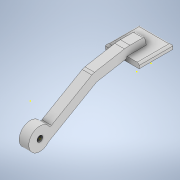
# Autodesk Inventor part: moving gripper
Saved by Autodesk Inventor 2021 (Build 250183000, 183)
## iProperties
Created: 2021-01-30
Part Number: moving gripper
Material: Generic
Document SubType Name: Modeling
Designer: josep
Density: 1 g/cm^3
Appearance: Default
Author: josep
Autodesk Inventor part; units mm, degrees
ref_plane "YZ Plane" through (0, 0, 0) normal (1, 0, 0) x (0, 1, 0)
ref_plane "XZ Plane" through (0, 0, 0) normal (0, 1, 0) x (-1, 0, 0)
ref_plane "XY Plane" through (0, 0, 0) normal (0, 0, 1) x (1, 0, 0)
sketch "Sketch1" plane through (0, 0, 0) normal (1, 0, 0) x (0, 1, 0)
  circle A0 centre (0, 0) radius 11.5
  line L0 (0, -11.5) -> (51.956, -11.5) construction
  line L1 (17.8954, -32.4957) -> (5.0882, -10.3131)
  line L2 (9.2351, -37.4957) -> (-7.2673, -8.9127)
  line L3 (9.2351, -37.4957) -> (21.6479, -58.9952)
  line L4 (30.3081, -53.9952) -> (17.8954, -32.4957)
  line L5 (21.6479, -58.9952) -> (28.9335, -100.3138)
  line L6 (21.6479, -58.9952) -> (73.6039, -58.9952) construction
  line L7 (30.6699, -110.1619) -> (40.4125, -107.9075)
  line L8 (40.4125, -107.9075) -> (31.3905, -56.7409)
  line L9 (40.4125, -107.9075) -> (92.3685, -107.9075) construction
  arc A1 (31.3905, -56.7409) -> (30.3081, -53.9952) centre (21.6479, -58.9952) ccw
  line L10 (28.9335, -110.4681) -> (30.6699, -110.1619)
  line L11 (28.9335, -100.3138) -> (28.9335, -110.4681)
  dimension "d0" = 23
  dimension "d4" = 10
  dimension "d7" = 10
  dimension "d9" = 100
  constraints: 24 end point, 5 point on circle, 3 horizontal, 2 centre point, 2 point on line, 1 coincident, 1 equal length, 1 parallel, 1 vertical
  measures "d0" diameter of A0
  measures "d4" distance of L1.start L2.start
  measures "d7" distance of L7.start L7.end
  measures "d9" angle of L9 L8
extrude "Extrusion1" add sketch "Sketch1" along normal blind 10
sketch "Sketch2" plane through (0, 28.9335, -110.4681) normal (0, -1, 0) x (1, 0, 0)
  line L0 (10, 51.4729) -> (10, 10.1543) projected
  line L1 (10, 10.1543) -> (10, 0) projected
  line L2 (10, 10.1543) -> (10, 0)
  line L3 (0, 0) -> (10, 0) projected
  line L4 (10, 0) -> (0, 0)
  line L5 (0, 10.1543) -> (10, 10.1543) projected
  line L6 (0, 0) -> (0, 10.1543)
  line L7 (0, 10.1543) -> (10, 10.1543)
  point P0 (0, 110.4681)
  constraints: 8 end point, 3 collinear, 1 perpendicular
extrude "Extrusion2" add sketch "Sketch2" along normal blind 5
sketch "Sketch3" plane through (10, 28.9335, -110.4681) normal (0, 0, -1) x (-1, 0, 0)
  point P0 (10, -28.9335)
sketch "Sketch4" plane through (10, 28.9335, -110.4681) normal (0, 0, -1) x (-1, 0, 0)
  line L0 (0, 0) -> (0, 1.7365) projected
  line L1 (10, 0) -> (10, 1.7365) projected
  line L2 (0, 0) -> (10, 0)
  line L3 (10, 0) -> (10, -5)
  line L4 (10, -5) -> (0, -5)
  line L5 (0, -5) -> (0, 0)
  point P0 (10, -28.9335)
  constraints: 8 end point, 3 perpendicular, 1 horizontal
extrude "Extrusion3" add sketch "Sketch4" along normal blind 15
sketch "Sketch5" plane through (10, 28.9335, -125.4681) normal (0, 0, -1) x (-1, 0, 0)
  point P0 (10, -28.9335)
sketch "Sketch6" plane through (10, 28.9335, -125.4681) normal (0, 0, -1) x (-1, 0, 0)
  line L0 (10, 0) -> (0, 0) projected
  line L1 (0, 0) -> (10, 0)
  line L2 (10, -5) -> (10, 0) projected
  line L3 (10, 0) -> (10, -5)
  line L4 (0, -5) -> (10, -5) projected
  line L5 (10, -5) -> (0, -5)
  line L6 (0, 0) -> (0, -5) projected
  line L7 (0, -5) -> (0, 0)
  point P0 (10, -28.9335)
  constraints: 8 end point, 2 collinear, 1 horizontal, 1 perpendicular
extrude "Extrusion4" add sketch "Sketch6" against normal blind 35
sketch "Sketch7" plane through (10, 0, 0) normal (1, 0, 0) x (0, 0, -1)
  point P0 (0, 0)
sketch "Sketch8" plane through (10, 0, 0) normal (1, 0, 0) x (0, 0, -1)
  line L0 (125.4681, 28.9335) -> (125.4681, 23.9335) projected
  line L1 (125.4681, 28.9335) -> (125.4681, 23.9335)
  line L2 (90.4681, 23.9335) -> (90.4681, 27.1974) projected
  line L3 (125.4681, 23.9335) -> (90.4681, 23.9335)
  line L4 (90.4681, 23.9335) -> (90.4681, 28.9335)
  line L5 (110.4681, 28.9335) -> (125.4681, 28.9335) projected
  line L6 (90.4681, 28.9335) -> (125.4681, 28.9335)
  point P0 (0, 0)
  constraints: 8 end point, 2 perpendicular, 1 collinear, 1 vertical
extrude "Extrusion5" add sketch "Sketch8" along normal blind 5
sketch "Sketch9" plane through (15, 0, 0) normal (1, 0, 0) x (0, 0, -1)
  line L0 (110.4681, 28.9335) -> (125.4681, 28.9335) projected
  line L1 (90.4681, 28.9335) -> (125.4681, 28.9335)
  line L2 (125.4681, 23.9335) -> (125.4681, 28.9335) projected
  line L3 (125.4681, 28.9335) -> (125.4681, 23.9335)
  line L4 (125.4681, 23.9335) -> (90.4681, 23.9335) projected
  line L5 (125.4681, 23.9335) -> (90.4681, 23.9335)
  line L6 (90.4681, 27.1974) -> (90.4681, 28.9335) projected
  line L7 (90.4681, 23.9335) -> (90.4681, 28.9335)
  point P0 (0, 0)
  constraints: 8 end point, 3 perpendicular, 1 collinear
extrude "Extrusion6" add sketch "Sketch9" along normal blind 10
sketch "Sketch10" plane through (0, 28.9335, -110.4681) normal (0, 1, 0) x (1, 0, 0)
  point P0 (0, -110.4681)
sketch "Sketch11" plane through (25, 0, 0) normal (1, 0, 0) x (0, 0, -1)
  line L0 (125.4681, 23.9335) -> (125.4681, 28.9335) projected
  line L1 (125.4681, 28.9335) -> (125.4681, 23.9335)
  line L2 (90.4681, 27.1974) -> (90.4681, 23.9335) projected
  line L3 (125.4681, 23.9335) -> (90.4681, 23.9335)
  line L4 (90.4681, 23.9335) -> (90.4681, 28.9335)
  line L5 (110.4681, 28.9335) -> (125.4681, 28.9335) projected
  line L6 (90.4681, 28.9335) -> (125.4681, 28.9335)
  point P0 (0, 0)
  constraints: 8 end point, 3 perpendicular, 1 vertical
extrude "Extrusion7" add sketch "Sketch11" against normal blind 35
sketch "Sketch12" plane through (0, 28.9335, -110.4681) normal (0, 1, 0) x (1, 0, 0)
  line L0 (10.067, -4.6635) -> (22.567, -4.6635)
  line L1 (22.567, -4.6635) -> (22.567, -20)
  line L2 (10, -20) -> (25, -20) projected
  line L3 (22.567, -20) -> (25, -20)
  line L4 (25, 15) -> (25, -20) projected
  line L5 (25, -20) -> (25, 15)
  line L6 (25, 15) -> (22.567, 15)
  line L7 (22.567, 15) -> (22.567, -4.6635)
  point P0 (0, -110.4681)
  dimension "d27" = 12.5
  constraints: 12 end point, 3 perpendicular, 2 point on line, 1 collinear, 1 horizontal
  measures "d27" distance of L0.start L0.end
extrude "Extrusion8" cut sketch "Sketch12" against normal blind 35
sketch "Sketch13" plane through (22.567, 28.9335, -90.4681) normal (1, 0, 0) x (0, 0, -1)
  line L0 (0, 0) -> (35, 0) projected
  line L1 (35, 0) -> (35, -5) projected
  line L2 (35, 0) -> (35, -5)
  line L3 (35, -5) -> (0, -5) projected
  line L4 (35, -5) -> (0, -5)
  line L5 (0, 0) -> (0, -1.7361) projected
  line L6 (0, -5) -> (0, 0)
  line L7 (0, 0) -> (35, 0)
  point P0 (-90.4681, -28.9335)
  constraints: 8 end point, 2 perpendicular, 1 collinear, 1 vertical
extrude "Extrusion9" add sketch "Sketch13" against normal blind 35
sketch "Sketch14" plane through (0, 0, 0) normal (-1, 0, 0) x (0, 0, 1)
  line L0 (-107.9075, 40.4125) -> (-56.7409, 31.3905) projected
  line L1 (-90.2619, 37.3011) -> (-108.6275, 37.3011)
  line L2 (-110.1619, 30.6699) -> (-107.9075, 40.4125) projected
  line L3 (-108.6275, 37.3011) -> (-107.9075, 40.4125)
  line L4 (-107.9075, 40.4125) -> (-90.2619, 37.3011)
  point P0 (0, 0)
  constraints: 6 end point, 2 point on line, 1 collinear, 1 horizontal
extrude "Extrusion10" cut sketch "Sketch14" against normal blind 35
sketch "Sketch15" plane through (0, 0, 0) normal (-1, 0, 0) x (0, 0, 1)
  line L0 (-90.2619, 37.3011) -> (-56.7409, 31.3905) projected
  line L1 (-108.6275, 37.3011) -> (-90.2619, 37.3011) projected
  arc A0 (-87.8441, 36.8748) -> (-93.5866, 37.3011) centre (-93.5866, -1.5878) ccw
  line L2 (-93.5866, 37.3011) -> (-90.2619, 37.3011)
  line L3 (-90.2619, 37.3011) -> (-87.8441, 36.8748)
  point P0 (0, 0)
  constraints: 4 end point, 2 collinear, 2 point on circle, 2 point on line, 1 centre point, 1 tangent
extrude "Extrusion11" cut sketch "Sketch15" against normal blind 35
sketch "Sketch16" plane through (0, 0, 0) normal (-1, 0, 0) x (0, 0, 1)
  point P0 (0, 0)
fillet "Fillet1" radius 2 1 edges at (5, 37.3011, -108.6275)
fillet "Fillet2" radius 2 4 edges at (5.067, 28.9335, -125.4681) (-12.433, 28.9335, -107.9681) (-6.2165, 28.9335, -90.4681) (22.567, 28.9335, -107.9681)
fillet "Fillet3" radius 2 1 edges at (5, 5.0882, -10.3131)
fillet "Fillet4" radius 2 2 edges at (5, 21.6479, -58.9952) (5, -7.2673, -8.9127)
sketch "Sketch17" plane through (10, 0, 0) normal (1, 0, 0) x (0, 0, -1)
  circle A0 centre (0, 0) radius 3
  dimension "d40" = 6
  constraints: 1 centre point, 1 coincident
  measures "d40" diameter of A0
extrude "Extrusion12" cut sketch "Sketch17" against normal blind 3.5
thread "Thread1" size "M6x1" class "6H" standard "ANSI Metric M Profile" full length
body "Solid1"
